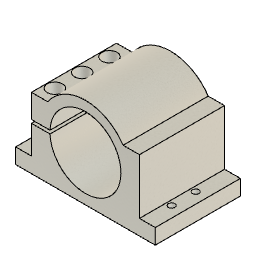
Spindle Clamp 65mm (Autodesk Fusion 360 design; units mm, degrees)
Autodesk Fusion 360 part; units mm, degrees
note: some values were not read from the file. Set by a fixed rule: which sketch regions a step uses.
sketch "Front" plane through (0, 0, 0) normal (0, 1, 0) x (1, 0, 0)
  line L0 (-75, -10) -> (75, -10) construction
  line L1 (-75, -24) -> (75, -24) construction
  line L2 (-75, -74.5651) -> (75, -74.5651) construction
  line L3 (-74, -51.5) -> (76, -51.5) construction
  circle A0 centre (1, -51.5) radius 32.5
  circle A1 centre (1, -51.5) radius 41.5
  line L4 (-48.5, 10) -> (-48.5, -85) construction
  line L5 (50.5, 10) -> (50.5, -85) construction
  line L6 (65, 10) -> (65, -25) construction
  line L7 (-63, 10) -> (-63, -25) construction
  line L8 (-33.5, -74.5651) -> (-48.5, -74.5651)
  line L9 (-48.5, -74.5651) -> (-48.5, -24)
  line L10 (-48.5, -24) -> (-63, -24)
  line L11 (-63, -24) -> (-63, -10)
  line L12 (-63, -10) -> (65, -10)
  line L13 (65, -10) -> (65, -24)
  line L14 (65, -24) -> (50.5, -24)
  line L15 (50.5, -24) -> (50.5, -74.5651)
  line L16 (50.5, -74.5651) -> (35.5, -74.5651)
  line L17 (-30, -53) -> (-51, -53)
  line L18 (-51, -53) -> (-51, -50)
  line L19 (-51, -50) -> (-30, -50)
  line L20 (-30, -50) -> (-30, -53)
  line L21 (-30, -53) -> (-51, -50) construction
  line L22 (-51, -53) -> (-30, -50) construction
  point P0 (-33.5, -74.5651)
  point P1 (35.5, -74.5651)
  point P2 (0.9773, -10)
  point P3 (-40.5, -51.5)
  dimension "d1" = 14
  dimension "d2" = 65
  dimension "d3" = 83
  dimension "d4" = 49.5
  dimension "d5" = 49.5
  dimension "d6" = 64
  dimension "d7" = 64
  dimension "d8" = 15
  dimension "d9" = 15
  dimension "d10" = 23.0651
  dimension "d14" = 14.5
  dimension "d15" = 3
  constraint horizontal L0
  constraint horizontal L1
  constraint parallel L1 L2
  constraint horizontal L3
  constraint midpoint L3 A0.centre
  constraint concentric A0 A1
  constraint perpendicular L2 L4
  constraint perpendicular L2 L5
  constraint perpendicular L3 L6
  constraint perpendicular L1 L7
  constraint coincident A1 P0
  constraint coincident L2 P0
  constraint coincident A1 P1
  constraint coincident L2 P1
  constraint coincident A1 P2
  constraint coincident P0 L8.start
  constraint coincident L4 L8.end
  constraint perpendicular L4 L8
  constraint coincident L4 L9.end
  constraint perpendicular L3 L9
  constraint coincident L7 L10.end
  constraint coincident L1 L10.end
  constraint perpendicular L7 L10
  constraint coincident L7 L11.end
  constraint coincident L0 L11.end
  constraint coincident L0 L12.end
  constraint coincident L6 L12.end
  constraint coincident L1 L13.end
  constraint coincident L6 L13.end
  constraint coincident L5 L14.end
  constraint coincident L1 L14.end
  constraint coincident L5 L15.end
  constraint coincident L2 L15.end
  constraint coincident P1 L16.end
  constraint perpendicular L17 L18
  constraint parallel L17 L19
  constraint parallel L18 L20
  constraint horizontal L17
  constraint coincident L21 P3
  constraint coincident L22 P3
  constraint coincident A1 P3
  constraint coincident L3 P3
  constraint tangent A1 L12
  measures "d1" distance of L0 L1
  measures "d2" diameter of A0
  measures "d3" diameter of A1
  measures "d4" distance of A0.centre L4
  measures "d5" distance of A0.centre L5
  measures "d6" distance of A0.centre L7
  measures "d7" distance of A0.centre L6
  measures "d8" distance of L4 P0
  measures "d9" distance of L5 P1
  measures "d10" distance of L2 L3
  measures "d14" distance of L4 L7
  measures "d15" distance of L17.end L18.end
extrude "Extrude1" add sketch "Front" along normal blind 78 contours A0 A1 L17 L19 | A1 L9 L10 L11 L12 L19 | A1 L8 L9 L17 | A1 L12 L13 L14 L15 L16 picked at (34.7953, -69.7412)
sketch "Top holes" plane through (0, 0, 74.5651) normal (0, 0, 1) x (-1, 0, 0)
  line L0 (48.5, 0) -> (33.5, 0)
  line L1 (33.5, 0) -> (33.5, -78)
  line L2 (33.5, -78) -> (48.5, -78)
  line L3 (48.5, -78) -> (48.5, 0)
  line L4 (41, -78) -> (41, 0) construction
  circle A0 centre (41, -39) radius 7
  circle A1 centre (41, -64) radius 7
  circle A2 centre (41, -14) radius 7
  circle A3 centre (41, -39) radius 4
  circle A4 centre (41, -64) radius 4
  circle A5 centre (41, -14) radius 4
  dimension "d18" = 14
  dimension "d19" = 14
  dimension "d20" = 14
  dimension "d21" = 25
  dimension "d22" = 25
  dimension "d23" = 8
  dimension "d24" = 8
  dimension "d25" = 8
  constraint midpoint L2 L4.start
  constraint midpoint L0 L4.end
  constraint midpoint L4 A0.centre
  constraint coincident L4 A1.centre
  constraint coincident L4 A2.centre
  constraint concentric A0 A3
  constraint concentric A1 A4
  constraint concentric A2 A5
  measures "d18" diameter of A0
  measures "d19" diameter of A1
  measures "d20" diameter of A2
  measures "d21" distance of A0.centre A1.centre
  measures "d22" distance of A0.centre A2.centre
  measures "d23" diameter of A3
  measures "d24" diameter of A4
  measures "d25" diameter of A5
extrude "Extrude2" cut sketch "Top holes" against normal blind 45 contours A4 | A5
extrude "Extrude5" cut sketch "Top holes" against normal blind 23 contours A3
extrude "Extrude3" cut sketch "Top holes" against normal blind 10 contours A0 | A1 | A2
sketch "Bottom holes" plane through (0, 0, 10) normal (0, 0, -1) x (1, 0, 0)
  line L0 (65, 0) -> (-63, 0)
  line L1 (-63, -78) -> (65, -78)
  line L2 (65, -78) -> (65, 0)
  line L3 (1, -78) -> (1, 0) construction
  line L4 (55, -47) -> (-53, -47) construction
  line L5 (-53, -47) -> (-53, -25) construction
  line L6 (-53, -25) -> (55, -25) construction
  line L7 (55, -25) -> (55, -47) construction
  line L8 (55, -47) -> (-53, -25) construction
  line L9 (-53, -47) -> (55, -25) construction
  circle A0 centre (-53, -25) radius 3
  circle A1 centre (-53, -47) radius 3
  circle A2 centre (55, -47) radius 3
  circle A3 centre (55, -25) radius 3
  line L10 (-63, 0) -> (-63, -78)
  point P0 (1, -36)
  dimension "d38" = 108
  dimension "d39" = 22
  dimension "d40" = 25
  dimension "d41" = 6
  dimension "d42" = 6
  dimension "d43" = 6
  dimension "d44" = 6
  constraint midpoint L1 L3.start
  constraint midpoint L0 L3.end
  constraint perpendicular L4 L5
  constraint parallel L4 L6
  constraint parallel L5 L7
  constraint horizontal L4
  constraint coincident L8 P0
  constraint coincident L9 P0
  constraint coincident L3 P0
  constraint coincident L5.end L6.start
  constraint coincident L4.end L5.start
  constraint coincident L4.start L7.end
  constraint coincident L6.end L7.start
  measures "d38" distance of L5.end L6.end
  measures "d39" distance of L4.end L5.end
  measures "d40" distance of L0 L6
  measures "d41" diameter of A0
  measures "d42" diameter of A1
  measures "d43" diameter of A2
  measures "d44" diameter of A3
extrude "Extrude4" cut sketch "Bottom holes" against normal through all contours A0 | A1 | A2 | A3
equation "d3 = d2 + 18 mm"
equation "d4 = ( 99 / 2 ) * 1 mm"
equation "d5 = d4"
equation "d7 = d6"
equation "d19 = d18"
equation "d20 = d18"
equation "d22 = d21"
equation "d24 = d23"
equation "d25 = d23"
equation "d42 = d41"
equation "d43 = d41"
equation "d44 = d41"
named bodies: "Clamp"
